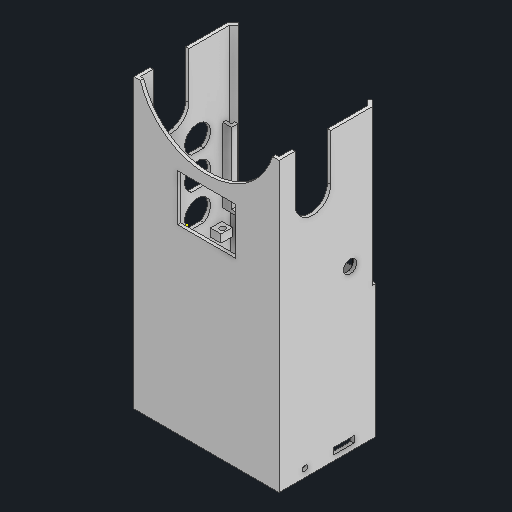
# Autodesk Inventor part: frame
Saved by Autodesk Inventor 2027.1 (Build 311270010, 270A)
## iProperties
Created: 2026-06-11
Part Number: frame
Material: Generic
Document SubType Name: Modeling
Designer: alexg
Density: 1 g/cm^3
Appearance: Default
Author: alexg
Autodesk Inventor part; units mm, degrees
sketch "Sketch1" plane through (0, 0, 0) normal (0, 1, 0) x (-1, 0, 0)
  line L0 (-45, 30) -> (45, 30)
  line L1 (45, 30) -> (45, -30)
  line L2 (45, -30) -> (-45, -30)
  line L3 (-45, -30) -> (-45, 30)
  line L4 (-45, 30) -> (45, -30) construction
  line L5 (45, 30) -> (-45, -30) construction
  line L6 (43, 28) -> (-43, 28)
  line L7 (-43, 28) -> (-43, -28)
  line L8 (-43, -28) -> (43, -28)
  line L9 (43, -28) -> (43, 28)
  point P0 (0, 0)
  dimension "d0" = 90
  dimension "d1" = 60
  dimension "d2" = 86
  dimension "d3" = 56
  dimension "d4" = 2
  dimension "d5" = 2
  constraints: 20 end point, 4 parallel, 2 horizontal, 2 midpoint, 2 perpendicular
  measures "d0" distance of L1.end L2.end
  measures "d1" distance of L0.end L1.end
  measures "d2" distance of L8.end L7.end
  measures "d3" distance of L7.end L6.end
  measures "d4" distance between parallel lines of L2 L8
  measures "d5" distance between parallel lines of L3 L7
extrude "Extrusion1" add sketch "Sketch1" along normal blind 44
sketch "Sketch2" plane through (0, 0, 0) normal (0, -1, 0) x (1, 0, 0)
  line L0 (-45, 30) -> (45, 30) projected
  line L1 (-45, 30) -> (45, 30)
  line L2 (45, 30) -> (45, -30)
  line L3 (45, -30) -> (-45, -30)
  line L4 (-45, -30) -> (-45, 30)
  point P0 (0, 0)
  constraints: 8 end point, 2 parallel, 1 horizontal, 1 perpendicular
extrude "Extrusion2" add sketch "Sketch2" along normal blind 2
sketch "Sketch3" plane through (45, 44, 30) normal (1, 0, 0) x (0, 0, -1)
  line L0 (0, -46) -> (0, 0) projected
  line L1 (0, -22.505) -> (53, -22.505)
  line L2 (2, 0) -> (58, 0) projected
  line L3 (2, -44) -> (58, -44) projected
  line L4 (51, 0) -> (53, 0)
  line L5 (53, -44) -> (51, -44)
  line L6 (53, -44) -> (55, -44)
  line L7 (55, -44) -> (55, 0)
  line L8 (55, 0) -> (53, 0)
  line L9 (53, 0) -> (53, -44)
  point P0 (30, -44)
  dimension "d10" = 53
  dimension "d12" = 2
  constraints: 14 end point, 4 point on line, 3 horizontal, 3 parallel, 1 perpendicular
  measures "d10" distance of L1.start L1.end
  measures "d12" distance of L8.end L7.end
extrude "Extrusion3" add sketch "Sketch3" against normal blind 90
sketch "Sketch4" plane through (45, 44, -30) normal (0, 0, -1) x (-1, 0, 0)
  line L0 (2, 0) -> (88, 0) projected
  line L1 (88, -44) -> (2, -44) projected
  line L2 (2, 0) -> (88, 0)
  line L3 (88, 0) -> (88, -44)
  line L4 (88, -44) -> (2, -44)
  line L5 (2, -44) -> (2, 0)
  point P0 (45, -44)
  point P1 (2, -44)
  constraints: 8 end point, 2 parallel, 1 horizontal, 1 perpendicular
extrude "Extrusion4" cut sketch "Sketch4" against normal blind 2
sketch "Sketch5" plane through (43, 44, -25) normal (0, 0, -1) x (-1, 0, 0)
  line L0 (0, 0) -> (86, 0) projected
  line L1 (5.5, 0) -> (80.5, 0)
  line L2 (80.5, 0) -> (80.5, -44)
  line L3 (80.5, -44) -> (5.5, -44)
  line L4 (5.5, -44) -> (5.5, 0)
  line L5 (0, -44) -> (0, 0) projected
  point P0 (43, -44)
  dimension "d17" = 75
  dimension "d18" = 44
  dimension "d19" = 5.5
  constraints: 8 end point, 2 parallel, 1 horizontal, 1 perpendicular, 1 point on line
  measures "d17" distance of L2.end L3.end
  measures "d18" distance of L1.end L2.end
  measures "d19" distance between parallel lines of L5 L4
extrude "Extrusion5" cut sketch "Sketch5" against normal blind 2
sketch "Sketch6" plane through (-43, 0, -23) normal (0, 0, 1) x (1, 0, 0)
  line L0 (5.5, 0) -> (5.5, 44) projected
  line L1 (5.5, 44) -> (3.5, 44)
  line L2 (3.5, 44) -> (3.5, 0)
  line L3 (3.5, 0) -> (5.5, 0)
  line L4 (5.5, 0) -> (5.5, 44)
  line L5 (86, 44) -> (80.5, 44) projected
  line L6 (80.5, 44) -> (82.5, 44)
  line L7 (82.5, 44) -> (82.5, 0)
  line L8 (82.5, 0) -> (80.5, 0)
  line L9 (80.5, 0) -> (80.5, 44)
  point P0 (43, 0)
  dimension "d22" = 2
  dimension "d23" = 44
  dimension "d24" = 2
  dimension "d25" = 44
  constraints: 16 end point, 4 parallel, 2 horizontal, 2 perpendicular
  measures "d22" distance of L3.end L2.end
  measures "d23" distance of L2.end L1.end
  measures "d24" distance of L7.end L8.end
  measures "d25" distance of L6.end L7.end
extrude "Extrusion6" add sketch "Sketch6" against normal blind 4
sketch "Sketch8" plane through (45, -2, -30) normal (0, 0, -1) x (-1, 0, 0)
  line L0 (90, 46) -> (0, 46) projected
  line L1 (0, 46) -> (7.5, 46)
  line L2 (7.5, 46) -> (7.5, 0)
  line L3 (7.5, 0) -> (0, 0)
  line L4 (0, 0) -> (0, 46)
  line L5 (89.984, 46) -> (82.484, 46)
  line L6 (82.484, 46) -> (82.484, 0)
  line L7 (82.484, 0) -> (89.984, 0)
  line L8 (89.984, 0) -> (89.984, 46)
  point P0 (45, 2)
  point P1 (7.5, 46)
  dimension "d30" = 7.5
  dimension "d31" = 46
  dimension "d32" = 7.5
  dimension "d33" = 46
  constraints: 16 end point, 4 parallel, 2 horizontal, 2 perpendicular, 1 point on line
  measures "d30" distance of L2.end L3.end
  measures "d31" distance of L1.end L2.end
  measures "d32" distance of L7.end L6.end
  measures "d33" distance of L6.end L5.end
extrude "Extrusion7" cut sketch "Sketch8" against normal blind 1
sketch "Sketch9" plane through (-45, 44, -30) normal (-1, 0, 0) x (0, 0, 1)
  line L0 (0, -46) -> (0, 0) projected
  line L1 (1, 0) -> (1, -44) projected
  line L2 (0, -46) -> (1, -46)
  line L3 (1, -46) -> (1, 0)
  line L4 (1, 0) -> (0, 0)
  line L5 (0, 0) -> (0, -46)
  point P0 (30, -44)
  constraints: 8 end point, 2 parallel, 1 horizontal, 1 perpendicular
extrude "Extrusion8" cut sketch "Sketch9" against normal blind 1
sketch "Sketch10" plane through (0, 0, 0) normal (0, 1, 0) x (1, 0, 0)
  line L0 (-43, 25) -> (-43, 29) projected
  line L1 (-43, 27) -> (43, 27)
  line L2 (43, 29) -> (43, 25) projected
  line L3 (-43, 27) -> (-40, 30)
  line L4 (-43, 27) -> (-38.7574, 27) construction
  line L5 (-40, 30) -> (-41.4142, 31.4142)
  line L6 (-41.4142, 31.4142) -> (-45, 27.8284)
  line L7 (-45, -30) -> (-45, 29) projected
  line L8 (43, 27) -> (40, 30)
  line L9 (43, 27) -> (47.2426, 27) construction
  line L10 (40, 30) -> (41.4142, 31.4142)
  line L11 (40, 30) -> (42, 30) construction
  line L12 (41.4142, 31.4142) -> (45, 27.8284)
  line L13 (45, 27.8284) -> (43.2071, 26.7929)
  line L14 (-45, 29) -> (-37.484, 29) projected
  line L15 (-43.8284, 29) -> (-43, 29)
  line L16 (-43, 27) -> (-43, 29)
  line L17 (43, 29) -> (37.5, 29) projected
  line L18 (43, 27) -> (43, 29)
  line L19 (43, 29) -> (43.8284, 29)
  point P0 (0, 0)
  dimension "d38" = 45
  dimension "d39" = 2
  dimension "d40" = 90
  dimension "d41" = 90
  dimension "d42" = 135
  dimension "d43" = 2
  dimension "d44" = 45
  dimension "d45" = 90
  constraints: 30 end point, 5 perpendicular, 4 point on line, 3 equal length, 3 horizontal, 2 midpoint, 1 collinear
  measures "d38" angle of L4 L3
  measures "d39" distance of L3.end L5.end
  measures "d40" angle of L5 L3
  measures "d41" angle of L6 L5
  measures "d42" angle of L9 L8
  measures "d43" distance of L8.end L10.end
  measures "d44" angle of L11 L10
  measures "d45" angle of L10 L12
extrude "Extrusion9" add sketch "Sketch10" along normal blind 44 and the other way blind 2 contours L0 L14 L3 | L14 L6 L5 L3 | L2 L8 L17 | L17 L8 L10 L12 L19
sketch "Sketch11" plane through (0, 44, 0) normal (0, 1, 0) x (1, 0, 0)
  line L0 (37.5, 29) -> (45, 29) projected
  line L1 (43.8203, 29) -> (45, 29)
  line L2 (43.8284, 29) -> (45, 27.8284)
  line L3 (45, -30) -> (45, 29) projected
  line L4 (43.8284, 29) -> (45.4853, 29) construction
  line L5 (45, 27.8284) -> (45, 29)
  line L6 (-43.8284, 29) -> (-45, 29) projected
  line L7 (-43.8284, 29) -> (-45, 27.8284)
  line L8 (-45, 29) -> (-45, -30) projected
  line L9 (-43.8284, 29) -> (-42.1716, 29) construction
  line L10 (-45, 27.8284) -> (-45, 29)
  line L11 (-45, 29) -> (-43.8284, 29)
  point P0 (0, 0)
  dimension "d48" = 45
  dimension "d49" = 135
  constraints: 16 end point, 3 point on line, 2 collinear, 2 equal length, 2 horizontal, 1 perpendicular, 1 vertical
  measures "d48" angle of L2 L4
  measures "d49" angle of L7 L9
extrude "Extrusion10" cut sketch "Sketch11" against normal blind 48
sketch "Sketch12" plane through (-37.484, -2, -30) normal (-1, 0, 0) x (0, 0, 1)
  line L0 (1, 0) -> (1, 2) projected
  line L1 (0, 0) -> (0, 2) projected
  line L2 (1, 2) -> (0, 2)
  line L3 (0, 2) -> (0, 0)
  line L4 (0, 0) -> (1, 0)
  line L5 (1, 0) -> (1, 2)
  point P0 (30, 2)
  constraints: 8 end point, 2 parallel, 1 horizontal, 1 perpendicular
extrude "Extrusion11" add sketch "Sketch12" along normal blind 4.5 and the other way blind 79
sketch "Sketch13" plane through (0, 0, 0) normal (0, 1, 0) x (1, 0, 0)
  circle A0 centre (0, 26.5) radius 2
  line L0 (-40, 30) -> (40, 30) projected
  point P0 (0, 0)
  point P1 (0, 30)
  dimension "d58" = 4
  dimension "d59" = 3.5
  constraints: 1 centre point, 1 midpoint
  measures "d58" diameter of A0
  measures "d59" distance of point (0, 30) A0.centre
extrude "Extrusion12" cut sketch "Sketch13" against normal blind 4.5
sketch "Sketch14" plane through (0, 44, 0) normal (0, 1, 0) x (1, 0, 0)
  line L0 (45, -30) -> (-45, -30) projected
  line L1 (45, -30) -> (-45, -30)
  line L2 (-45, -30) -> (-45, 27.8284)
  line L3 (-41.4142, 31.4142) -> (-40, 30) projected
  line L4 (-45, 27.8284) -> (-41.4142, 31.4142)
  line L5 (-41.4142, 31.4142) -> (-40, 30)
  line L6 (-43, 27) -> (-40, 30)
  line L7 (43, -28) -> (-43, -28) projected
  line L8 (-43, 27) -> (-43, -28)
  line L9 (43, -28) -> (43, 27)
  line L10 (45, 27.8284) -> (45, -30) projected
  line L11 (40, 30) -> (43, 27) projected
  line L12 (43, 27) -> (40, 30)
  line L13 (40, 30) -> (41.4142, 31.4142) projected
  line L14 (40, 30) -> (41.4142, 31.4142)
  line L15 (41.4142, 31.4142) -> (45, 27.8284)
  point P0 (0, 0)
  constraints: 20 end point, 5 perpendicular, 3 collinear, 1 parallel, 1 vertical
extrude "Extrusion13" add sketch "Sketch14" along normal blind 50
sketch "Sketch15" plane through (43, 0, 28) normal (0, 0, -1) x (-1, 0, 0)
  circle A0 centre (43, 107) radius 43
  line L0 (0, 94) -> (86, 94) projected
  point P0 (43, 0)
  point P1 (83.9878, 94)
  point P2 (2.0122, 94)
  dimension "d64" = 86
  dimension "d65" = 13
  constraints: 1 centre point
  measures "d64" diameter of A0
  measures "d65" distance from line of L0 A0.centre
extrude "Extrusion14" cut sketch "Sketch15" against normal blind 16 contours L0 A0 picked at (43, 84)
sketch "Sketch16" plane through (-43, 0, 28) normal (1, 0, 0) x (0, 0, -1)
  circle A0 centre (19, 65) radius 11
  line L0 (0, 94) -> (55, 94) projected
  line L1 (0, 94) -> (0, 64) projected
  line L2 (8, 65) -> (8, 94)
  line L3 (30, 65) -> (30, 94)
  point P0 (28, 0)
  dimension "d68" = 22
  dimension "d69" = 29
  dimension "d70" = 19
  constraints: 4 end point, 2 perpendicular, 2 point on circle, 2 point on line, 2 tangent, 1 centre point
  measures "d68" diameter of A0
  measures "d69" distance from line of L0 A0.centre
  measures "d70" distance from line of L1 A0.centre
sketch "Sketch17" plane through (43, 0, -23) normal (-1, 0, 0) x (0, 0, 1)
  circle A0 centre (32, 65) radius 11
  line L0 (-4, 94) -> (51, 94) projected
  line L1 (51, 0) -> (51, 94) projected
  line L2 (43, 65) -> (43, 94)
  line L3 (43, 65) -> (72, 65) construction
  line L4 (21, 65) -> (21, 94)
  line L5 (21, 65) -> (50, 65) construction
  line L6 (21, 94) -> (43, 94)
  point P0 (23, 0)
  dimension "d71" = 22
  dimension "d72" = 29
  dimension "d73" = 19
  dimension "d74" = 90
  dimension "d75" = 90
  constraints: 10 end point, 2 horizontal, 2 perpendicular, 2 point on circle, 2 point on line, 1 centre point, 1 collinear
  measures "d71" diameter of A0
  measures "d72" distance from line of L0 A0.centre
  measures "d73" distance from line of L1 A0.centre
  measures "d74" angle of L3 L2
  measures "d75" angle of L5 L4
extrude "Extrusion15" cut sketch "Sketch17" against normal blind 16
extrude "Extrusion16" cut sketch "Sketch16" against normal blind 16
sketch "Sketch18" plane through (-43, 0, 28) normal (1, 0, 0) x (0, 0, -1)
  point P0 (28, 0)
chamfer "Chamfer1" distance 2 angle 45 3 edges at (0, 0, 28) (43, 0, 2.5) (-43, 0, 2.5)
ref_plane "Work Plane1" through (0, -2, 0) normal (0, 1, 0) x (-1, 0, 0)
sketch "Enc_OpenFloor sketch" plane through (0, -2, 0) normal (0, 1, 0) x (-1, 0, 0)
  line L0 (43, -23) -> (-43, -23)
  line L1 (-43, -23) -> (-43, 28)
  line L2 (-43, 28) -> (43, 28)
  line L3 (43, 28) -> (43, -23)
  constraints: 8 end point, 2 parallel, 1 horizontal, 1 perpendicular
extrude "Enc_OpenFloor" cut sketch "Enc_OpenFloor sketch" along normal blind 4
ref_plane "Work Plane2" through (0, -2, 0) normal (0, 1, 0) x (-1, 0, 0)
sketch "Enc_Skirt sketch" plane through (0, -2, 0) normal (0, 1, 0) x (-1, 0, 0)
  line L0 (45, -30) -> (-45, -30)
  line L1 (-45, -30) -> (-45, 30)
  line L2 (-45, 30) -> (45, 30)
  line L3 (45, 30) -> (45, -30)
  line L4 (43, -28) -> (-43, -28)
  line L5 (-43, -28) -> (-43, 28)
  line L6 (-43, 28) -> (43, 28)
  line L7 (43, 28) -> (43, -28)
  constraints: 16 end point, 4 parallel, 2 horizontal, 2 perpendicular
extrude "Enc_Skirt" add sketch "Enc_Skirt sketch" against normal blind 82.37
ref_plane "Work Plane3" through (0, -2, 0) normal (0, 1, 0) x (-1, 0, 0)
sketch "Enc_ScrewAccessGroove sketch" plane through (0, -2, 0) normal (0, 1, 0) x (-1, 0, 0)
  line L0 (3, -29) -> (-3, -29)
  line L1 (-3, -29) -> (-3, -28)
  line L2 (-3, -28) -> (3, -28)
  line L3 (3, -28) -> (3, -29)
  constraints: 8 end point, 2 parallel, 1 horizontal, 1 perpendicular
extrude "Enc_ScrewAccessGroove" cut sketch "Enc_ScrewAccessGroove sketch" against normal blind 82.37
ref_plane "Work Plane4" through (0, -14, 0) normal (0, 1, 0) x (-1, 0, 0)
sketch "Enc_SelenoHangers sketch" plane through (0, -14, 0) normal (0, 1, 0) x (-1, 0, 0)
  line L0 (-36.5, 20.5) -> (-43, 20.5)
  line L1 (-43, 20.5) -> (-43, 28)
  line L2 (-43, 28) -> (-36.5, 28)
  line L3 (-36.5, 28) -> (-36.5, 20.5)
  line L4 (-36.5, -22.5) -> (-43, -22.5)
  line L5 (-43, -22.5) -> (-43, -15.5)
  line L6 (-43, -15.5) -> (-36.5, -15.5)
  line L7 (-36.5, -15.5) -> (-36.5, -22.5)
  line L8 (43, 20.5) -> (36.5, 20.5)
  line L9 (36.5, 20.5) -> (36.5, 28)
  line L10 (36.5, 28) -> (43, 28)
  line L11 (43, 28) -> (43, 20.5)
  line L12 (43, -22.5) -> (36.5, -22.5)
  line L13 (36.5, -22.5) -> (36.5, -15.5)
  line L14 (36.5, -15.5) -> (43, -15.5)
  line L15 (43, -15.5) -> (43, -22.5)
  constraints: 32 end point, 8 parallel, 4 horizontal, 4 perpendicular
extrude "Enc_SelenoHangers" add sketch "Enc_SelenoHangers sketch" along normal blind 5
ref_plane "Work Plane5" through (0, -14, 0) normal (0, 1, 0) x (-1, 0, 0)
sketch "Enc_SelenoInsertHoles sketch" plane through (0, -14, 0) normal (0, 1, 0) x (-1, 0, 0)
  circle A0 centre (-39, 24) radius 1.75
  circle A1 centre (-39, -19) radius 1.75
  circle A2 centre (39, 24) radius 1.75
  circle A3 centre (39, -19) radius 1.75
  constraints: 4 centre point
extrude "Enc_SelenoInsertHoles" cut sketch "Enc_SelenoInsertHoles sketch" along normal blind 5
ref_plane "Work Plane6" through (-46, 0, 0) normal (1, 0, 0) x (0, 1, 0)
sketch "Enc_ButtonHoles sketch" plane through (-46, 0, 0) normal (1, 0, 0) x (0, 1, 0)
  arc A0 (36, -11.373) -> (36, -3.627) centre (43, -7.5) ccw
  line L0 (36, -3.627) -> (36, -11.373)
  arc A1 (36, 8.627) -> (36, 16.373) centre (43, 12.5) ccw
  line L1 (36, 16.373) -> (36, 8.627)
  arc A2 (16, -11.373) -> (16, -3.627) centre (23, -7.5) ccw
  line L2 (16, -3.627) -> (16, -11.373)
  arc A3 (16, 8.627) -> (16, 16.373) centre (23, 12.5) ccw
  line L3 (16, 16.373) -> (16, 8.627)
  arc A4 (-4, -11.373) -> (-4, -3.627) centre (3, -7.5) ccw
  line L4 (-4, -3.627) -> (-4, -11.373)
  arc A5 (-4, 8.627) -> (-4, 16.373) centre (3, 12.5) ccw
  line L5 (-4, 16.373) -> (-4, 8.627)
  constraints: 12 end point, 12 point on circle, 6 centre point
extrude "Enc_ButtonHoles" cut sketch "Enc_ButtonHoles sketch" along normal blind 4
ref_plane "Work Plane7" through (46, 0, 0) normal (1, 0, 0) x (0, 1, 0)
sketch "Enc_PowerSocketHole sketch" plane through (46, 0, 0) normal (1, 0, 0) x (0, 1, 0)
  circle A0 centre (15, -14) radius 4.1
  constraints: 1 centre point
extrude "Enc_PowerSocketHole" cut sketch "Enc_PowerSocketHole sketch" against normal blind 4
ref_plane "Work Plane8" through (0, 0, 31) normal (0, 0, 1) x (1, 0, 0)
sketch "Enc_ScreenWindow sketch" plane through (0, 0, 31) normal (0, 0, 1) x (1, 0, 0)
  line L0 (-18, 28) -> (18, 28)
  line L1 (18, 28) -> (18, 57)
  line L2 (18, 57) -> (-18, 57)
  line L3 (-18, 57) -> (-18, 28)
  constraints: 8 end point, 2 parallel, 1 horizontal, 1 perpendicular
extrude "Enc_ScreenWindow" cut sketch "Enc_ScreenWindow sketch" against normal blind 4
ref_plane "Work Plane9" through (0, 0, -31) normal (0, 0, 1) x (1, 0, 0)
sketch "Enc_PiUSBCutout sketch" plane through (0, 0, -31) normal (0, 0, 1) x (1, 0, 0)
  line L0 (-5.93, -82.79) -> (6.07, -82.79)
  line L1 (6.07, -82.79) -> (6.07, -74.29)
  line L2 (6.07, -74.29) -> (-5.93, -74.29)
  line L3 (-5.93, -74.29) -> (-5.93, -82.79)
  constraints: 8 end point, 2 parallel, 1 horizontal, 1 perpendicular
extrude "Enc_PiUSBCutout" cut sketch "Enc_PiUSBCutout sketch" along normal blind 4
ref_plane "Work Plane10" through (46, 0, 0) normal (1, 0, 0) x (0, 1, 0)
sketch "Enc_PiSDCardSlot sketch" plane through (46, 0, 0) normal (1, 0, 0) x (0, 1, 0)
  line L0 (-81.07, -16.6) -> (-77.07, -16.6)
  line L1 (-77.07, -16.6) -> (-77.07, -3.6)
  line L2 (-77.07, -3.6) -> (-81.07, -3.6)
  line L3 (-81.07, -3.6) -> (-81.07, -16.6)
  constraints: 8 end point, 2 parallel, 1 horizontal, 1 perpendicular
extrude "Enc_PiSDCardSlot" cut sketch "Enc_PiSDCardSlot sketch" against normal blind 4
ref_plane "Work Plane11" through (-46, 0, 0) normal (1, 0, 0) x (0, 1, 0)
sketch "Enc_BaseScrewHolesL sketch" plane through (-46, 0, 0) normal (1, 0, 0) x (0, 1, 0)
  circle A0 centre (-79.37, -12) radius 1.7
  circle A1 centre (-79.37, 14) radius 1.7
  constraints: 2 centre point
extrude "Enc_BaseScrewHolesL" cut sketch "Enc_BaseScrewHolesL sketch" along normal blind 4
ref_plane "Work Plane12" through (46, 0, 0) normal (1, 0, 0) x (0, 1, 0)
sketch "Enc_BaseScrewHolesR sketch" plane through (46, 0, 0) normal (1, 0, 0) x (0, 1, 0)
  circle A0 centre (-79.37, 14) radius 1.7
  constraints: 1 centre point
extrude "Enc_BaseScrewHolesR" cut sketch "Enc_BaseScrewHolesR sketch" against normal blind 4
ref_plane "Work Plane13" through (0, 0, -31) normal (0, 0, 1) x (1, 0, 0)
sketch "Enc_BaseScrewHolesB sketch" plane through (0, 0, -31) normal (0, 0, 1) x (1, 0, 0)
  circle A0 centre (-34, -79.37) radius 1.7
  constraints: 1 centre point
extrude "Enc_BaseScrewHolesB" cut sketch "Enc_BaseScrewHolesB sketch" along normal blind 4
ref_plane "Work Plane14" through (0, 0, 28) normal (0, 0, 1) x (1, 0, 0)
sketch "Enc_ScreenBosses sketch" plane through (0, 0, 28) normal (0, 0, 1) x (1, 0, 0)
  circle A0 centre (-26.935, 27) radius 1.9
  circle A1 centre (23.995, 27) radius 1.9
  circle A2 centre (-26.935, 58) radius 1.9
  circle A3 centre (23.995, 58) radius 1.9
  constraints: 4 centre point
extrude "Enc_ScreenBosses" add sketch "Enc_ScreenBosses sketch" against normal blind 2.6
ref_plane "Work Plane15" through (0, 0, 25.4) normal (0, 0, 1) x (1, 0, 0)
sketch "Enc_ScreenPilotHoles sketch" plane through (0, 0, 25.4) normal (0, 0, 1) x (1, 0, 0)
  circle A0 centre (-26.935, 27) radius 0.8
  circle A1 centre (23.995, 27) radius 0.8
  circle A2 centre (-26.935, 58) radius 0.8
  circle A3 centre (23.995, 58) radius 0.8
  constraints: 4 centre point
extrude "Enc_ScreenPilotHoles" cut sketch "Enc_ScreenPilotHoles sketch" along normal blind 4
body "Solid1"
